Autodesk Fusion 360 part; units mm, degrees
(part 12 of 12)
  arc A2532 (-131.6306, -63.5725) -> (-131.9356, -63.5725) centre (-131.7831, -63.5725) ccw
  arc A2533 (-131.9356, -63.5725) -> (-131.6306, -63.5725) centre (-131.7831, -63.5725) ccw
  arc A2534 (-71.9356, -63.5296) -> (-71.6306, -63.5296) centre (-71.7831, -63.5296) ccw
  arc A2535 (-71.6306, -63.5296) -> (-71.9356, -63.5296) centre (-71.7831, -63.5296) ccw
  arc A2536 (1.2955, -62.3231) -> (0.9905, -62.3231) centre (1.143, -62.3231) ccw
  arc A2537 (0.9905, -62.3231) -> (1.2955, -62.3231) centre (1.143, -62.3231) ccw
  arc A2538 (40.3074, -119.5512) -> (40.0024, -119.5512) centre (40.1549, -119.5512) ccw
  arc A2539 (40.0024, -119.5512) -> (40.3074, -119.5512) centre (40.1549, -119.5512) ccw
  arc A2540 (1.4833, -125.0963) -> (1.7883, -125.0963) centre (1.6358, -125.0963) ccw
  arc A2541 (1.7883, -125.0963) -> (1.4833, -125.0963) centre (1.6358, -125.0963) ccw
  arc A2542 (81.1583, -116.9472) -> (80.8533, -116.9472) centre (81.0058, -116.9472) ccw
  arc A2543 (80.8533, -116.9472) -> (81.1583, -116.9472) centre (81.0058, -116.9472) ccw
  arc A2544 (81.5772, 15.3665) -> (81.8822, 15.3665) centre (81.7297, 15.3665) ccw
  arc A2545 (81.8822, 15.3665) -> (81.5772, 15.3665) centre (81.7297, 15.3665) ccw
  arc A2546 (78.2397, -115.5227) -> (78.5447, -115.5227) centre (78.3922, -115.5227) ccw
  arc A2547 (78.5447, -115.5227) -> (78.2397, -115.5227) centre (78.3922, -115.5227) ccw
  arc A2548 (77.7039, -117.8524) -> (77.3989, -117.8524) centre (77.5514, -117.8524) ccw
  arc A2549 (77.3989, -117.8524) -> (77.7039, -117.8524) centre (77.5514, -117.8524) ccw
  arc A2550 (76.3501, -85.9792) -> (76.0451, -85.9792) centre (76.1976, -85.9792) ccw
  arc A2551 (76.0451, -85.9792) -> (76.3501, -85.9792) centre (76.1976, -85.9792) ccw
  arc A2552 (79.0501, -85.9792) -> (78.7451, -85.9792) centre (78.8976, -85.9792) ccw
  arc A2553 (78.7451, -85.9792) -> (79.0501, -85.9792) centre (78.8976, -85.9792) ccw
  arc A2554 (77.6836, -112.2817) -> (77.3786, -112.2817) centre (77.5311, -112.2817) ccw
  arc A2555 (77.3786, -112.2817) -> (77.6836, -112.2817) centre (77.5311, -112.2817) ccw
  arc A2556 (73.7743, -112.2817) -> (74.0793, -112.2817) centre (73.9268, -112.2817) ccw
  arc A2557 (74.0793, -112.2817) -> (73.7743, -112.2817) centre (73.9268, -112.2817) ccw
  arc A2558 (73.7743, -116.9995) -> (74.0793, -116.9995) centre (73.9268, -116.9995) ccw
  arc A2559 (74.0793, -116.9995) -> (73.7743, -116.9995) centre (73.9268, -116.9995) ccw
  arc A2560 (44.737, -78.1687) -> (45.042, -78.1687) centre (44.8895, -78.1687) ccw
  arc A2561 (45.042, -78.1687) -> (44.737, -78.1687) centre (44.8895, -78.1687) ccw
  arc A2562 (62.8957, -60.3089) -> (62.5907, -60.3089) centre (62.7432, -60.3089) ccw
  arc A2563 (62.5907, -60.3089) -> (62.8957, -60.3089) centre (62.7432, -60.3089) ccw
  arc A2564 (58.0289, -64.1397) -> (58.3339, -64.1397) centre (58.1814, -64.1397) ccw
  arc A2565 (58.3339, -64.1397) -> (58.0289, -64.1397) centre (58.1814, -64.1397) ccw
  arc A2566 (25.4347, -33.4412) -> (25.7398, -33.4412) centre (25.5872, -33.4412) ccw
  arc A2567 (25.7398, -33.4412) -> (25.4347, -33.4412) centre (25.5872, -33.4412) ccw
  arc A2568 (54.4271, -5.5405) -> (54.7321, -5.5405) centre (54.5796, -5.5405) ccw
  arc A2569 (54.7321, -5.5405) -> (54.4271, -5.5405) centre (54.5796, -5.5405) ccw
  arc A2570 (43.932, 19.9916) -> (43.627, 19.9916) centre (43.7795, 19.9916) ccw
  arc A2571 (43.627, 19.9916) -> (43.932, 19.9916) centre (43.7795, 19.9916) ccw
  arc A2572 (30.1477, 19.9916) -> (29.8427, 19.9916) centre (29.9952, 19.9916) ccw
  arc A2573 (29.8427, 19.9916) -> (30.1477, 19.9916) centre (29.9952, 19.9916) ccw
  arc A2574 (54.9582, -6.8923) -> (54.6532, -6.8923) centre (54.8057, -6.8923) ccw
  arc A2575 (54.6532, -6.8923) -> (54.9582, -6.8923) centre (54.8057, -6.8923) ccw
  arc A2576 (19.2295, -34.9096) -> (18.9245, -34.9096) centre (19.077, -34.9096) ccw
  arc A2577 (18.9245, -34.9096) -> (19.2295, -34.9096) centre (19.077, -34.9096) ccw
  arc A2578 (48.9839, -36.415) -> (49.2889, -36.415) centre (49.1364, -36.415) ccw
  arc A2579 (49.2889, -36.415) -> (48.9839, -36.415) centre (49.1364, -36.415) ccw
  arc A2580 (-161.9915, -49.4031) -> (-161.6865, -49.4031) centre (-161.839, -49.4031) ccw
  arc A2581 (-161.6865, -49.4031) -> (-161.9915, -49.4031) centre (-161.839, -49.4031) ccw
  arc A2582 (-178.5523, -46.4056) -> (-178.2473, -46.4056) centre (-178.3998, -46.4056) ccw
  arc A2583 (-178.2473, -46.4056) -> (-178.5523, -46.4056) centre (-178.3998, -46.4056) ccw
  arc A2584 (80.1576, -110.2962) -> (79.8526, -110.2962) centre (80.0051, -110.2962) ccw
  arc A2585 (79.8526, -110.2962) -> (80.1576, -110.2962) centre (80.0051, -110.2962) ccw
  arc A2586 (51.8899, -115.889) -> (51.5849, -115.889) centre (51.7374, -115.889) ccw
  arc A2587 (51.5849, -115.889) -> (51.8899, -115.889) centre (51.7374, -115.889) ccw
  arc A2588 (80.9549, -115.2316) -> (81.2599, -115.2316) centre (81.1074, -115.2316) ccw
  arc A2589 (81.2599, -115.2316) -> (80.9549, -115.2316) centre (81.1074, -115.2316) ccw
  arc A2590 (-184.9643, 17.1631) -> (-185.2693, 17.1631) centre (-185.1168, 17.1631) ccw
  arc A2591 (-185.2693, 17.1631) -> (-184.9643, 17.1631) centre (-185.1168, 17.1631) ccw
  arc A2592 (-169.0275, 17.1631) -> (-168.7225, 17.1631) centre (-168.875, 17.1631) ccw
  arc A2593 (-168.7225, 17.1631) -> (-169.0275, 17.1631) centre (-168.875, 17.1631) ccw
  arc A2594 (45.3849, 16.3147) -> (45.0799, 16.3147) centre (45.2324, 16.3147) ccw
  arc A2595 (45.0799, 16.3147) -> (45.3849, 16.3147) centre (45.2324, 16.3147) ccw
  arc A2596 (68.1408, -38.6081) -> (67.8358, -38.6081) centre (67.9883, -38.6081) ccw
  arc A2597 (67.8358, -38.6081) -> (68.1408, -38.6081) centre (67.9883, -38.6081) ccw
  arc A2598 (-155.29, 20.8895) -> (-155.595, 20.8895) centre (-155.4425, 20.8895) ccw
  arc A2599 (-155.595, 20.8895) -> (-155.29, 20.8895) centre (-155.4425, 20.8895) ccw
  arc A2600 (-124.4523, 23.0592) -> (-124.7573, 23.0592) centre (-124.6048, 23.0592) ccw
  arc A2601 (-124.7573, 23.0592) -> (-124.4523, 23.0592) centre (-124.6048, 23.0592) ccw
  arc A2602 (-121.9328, -27.0211) -> (-122.2378, -27.0211) centre (-122.0853, -27.0211) ccw
  arc A2603 (-122.2378, -27.0211) -> (-121.9328, -27.0211) centre (-122.0853, -27.0211) ccw
  arc A2604 (72.8017, -37.3381) -> (72.4967, -37.3381) centre (72.6492, -37.3381) ccw
  arc A2605 (72.4967, -37.3381) -> (72.8017, -37.3381) centre (72.6492, -37.3381) ccw
  arc A2606 (-90.8551, -43.2421) -> (-91.1601, -43.2421) centre (-91.0076, -43.2421) ccw
  arc A2607 (-91.1601, -43.2421) -> (-90.8551, -43.2421) centre (-91.0076, -43.2421) ccw
  arc A2608 (-88.1108, -46.4056) -> (-87.8058, -46.4056) centre (-87.9583, -46.4056) ccw
  arc A2609 (-87.8058, -46.4056) -> (-88.1108, -46.4056) centre (-87.9583, -46.4056) ccw
  arc A2610 (-67.864, 28.6035) -> (-67.559, 28.6035) centre (-67.7115, 28.6035) ccw
  arc A2611 (-67.559, 28.6035) -> (-67.864, 28.6035) centre (-67.7115, 28.6035) ccw
  arc A2612 (-38.6382, 27.985) -> (-38.9432, 27.985) centre (-38.7907, 27.985) ccw
  arc A2613 (-38.9432, 27.985) -> (-38.6382, 27.985) centre (-38.7907, 27.985) ccw
  arc A2614 (36.2051, -47.3741) -> (35.9001, -47.3741) centre (36.0526, -47.3741) ccw
  arc A2615 (35.9001, -47.3741) -> (36.2051, -47.3741) centre (36.0526, -47.3741) ccw
  arc A2616 (-37.7898, 28.636) -> (-37.4848, 28.636) centre (-37.6373, 28.636) ccw
  arc A2617 (-37.4848, 28.636) -> (-37.7898, 28.636) centre (-37.6373, 28.636) ccw
  arc A2618 (-17.3712, 28.0457) -> (-17.0662, 28.0457) centre (-17.2187, 28.0457) ccw
  arc A2619 (-17.0662, 28.0457) -> (-17.3712, 28.0457) centre (-17.2187, 28.0457) ccw
  arc A2620 (42.4739, -51.3081) -> (42.7789, -51.3081) centre (42.6264, -51.3081) ccw
  arc A2621 (42.7789, -51.3081) -> (42.4739, -51.3081) centre (42.6264, -51.3081) ccw
  arc A2622 (49.9036, -50.0381) -> (49.5986, -50.0381) centre (49.7511, -50.0381) ccw
  arc A2623 (49.5986, -50.0381) -> (49.9036, -50.0381) centre (49.7511, -50.0381) ccw
  arc A2624 (21.1086, 22.5339) -> (20.8036, 22.5339) centre (20.9561, 22.5339) ccw
  arc A2625 (20.8036, 22.5339) -> (21.1086, 22.5339) centre (20.9561, 22.5339) ccw
  arc A2626 (-115.7443, 22.5339) -> (-115.4393, 22.5339) centre (-115.5918, 22.5339) ccw
  arc A2627 (-115.4393, 22.5339) -> (-115.7443, 22.5339) centre (-115.5918, 22.5339) ccw
  arc A2628 (-117.869, 5.461) -> (-117.564, 5.461) centre (-117.7165, 5.461) ccw
  arc A2629 (-117.564, 5.461) -> (-117.869, 5.461) centre (-117.7165, 5.461) ccw
  arc A2630 (-178.0136, 5.461) -> (-177.7086, 5.461) centre (-177.8611, 5.461) ccw
  arc A2631 (-177.7086, 5.461) -> (-178.0136, 5.461) centre (-177.8611, 5.461) ccw
  arc A2632 (68.1307, -73.8407) -> (67.8257, -73.8407) centre (67.9782, -73.8407) ccw
  arc A2633 (67.8257, -73.8407) -> (68.1307, -73.8407) centre (67.9782, -73.8407) ccw
  arc A2634 (76.4972, -73.8407) -> (76.8022, -73.8407) centre (76.6497, -73.8407) ccw
  arc A2635 (76.8022, -73.8407) -> (76.4972, -73.8407) centre (76.6497, -73.8407) ccw
  arc A2636 (77.8462, -114.937) -> (77.5412, -114.937) centre (77.6937, -114.937) ccw
  arc A2637 (77.5412, -114.937) -> (77.8462, -114.937) centre (77.6937, -114.937) ccw
  arc A2638 (-116.4804, -5.8308) -> (-116.1754, -5.8308) centre (-116.3279, -5.8308) ccw
  arc A2639 (-116.1754, -5.8308) -> (-116.4804, -5.8308) centre (-116.3279, -5.8308) ccw
  arc A2640 (-90.2442, -94.2073) -> (-89.9392, -94.2073) centre (-90.0917, -94.2073) ccw
  arc A2641 (-89.9392, -94.2073) -> (-90.2442, -94.2073) centre (-90.0917, -94.2073) ccw
  arc A2642 (-155.29, -9.1105) -> (-155.595, -9.1105) centre (-155.4425, -9.1105) ccw
  arc A2643 (-155.595, -9.1105) -> (-155.29, -9.1105) centre (-155.4425, -9.1105) ccw
  arc A2644 (-124.5213, -6.8494) -> (-124.2163, -6.8494) centre (-124.3688, -6.8494) ccw
  arc A2645 (-124.2163, -6.8494) -> (-124.5213, -6.8494) centre (-124.3688, -6.8494) ccw
  arc A2646 (-148.7294, -6.4173) -> (-149.0344, -6.4173) centre (-148.8819, -6.4173) ccw
  arc A2647 (-149.0344, -6.4173) -> (-148.7294, -6.4173) centre (-148.8819, -6.4173) ccw
  arc A2648 (52.3113, -22.0432) -> (52.6163, -22.0432) centre (52.4638, -22.0432) ccw
  arc A2649 (52.6163, -22.0432) -> (52.3113, -22.0432) centre (52.4638, -22.0432) ccw
  arc A2650 (68.3591, -95.077) -> (68.6641, -95.077) centre (68.5116, -95.077) ccw
  arc A2651 (68.6641, -95.077) -> (68.3591, -95.077) centre (68.5116, -95.077) ccw
  arc A2652 (-126.5478, 2.5314) -> (-126.8528, 2.5314) centre (-126.7003, 2.5314) ccw
  arc A2653 (-126.8528, 2.5314) -> (-126.5478, 2.5314) centre (-126.7003, 2.5314) ccw
  arc A2654 (-95.8876, 2.5314) -> (-95.5826, 2.5314) centre (-95.7351, 2.5314) ccw
  arc A2655 (-95.5826, 2.5314) -> (-95.8876, 2.5314) centre (-95.7351, 2.5314) ccw
  arc A2656 (72.4233, -32.4915) -> (72.1183, -32.4915) centre (72.2708, -32.4915) ccw
  arc A2657 (72.1183, -32.4915) -> (72.4233, -32.4915) centre (72.2708, -32.4915) ccw
  arc A2658 (-64.483, -13.1039) -> (-64.788, -13.1039) centre (-64.6355, -13.1039) ccw
  arc A2659 (-64.788, -13.1039) -> (-64.483, -13.1039) centre (-64.6355, -13.1039) ccw
  arc A2660 (-30.2044, -7.1473) -> (-30.5094, -7.1473) centre (-30.3569, -7.1473) ccw
  arc A2661 (-30.5094, -7.1473) -> (-30.2044, -7.1473) centre (-30.3569, -7.1473) ccw
  arc A2662 (-51.1939, -97.062) -> (-50.8889, -97.062) centre (-51.0414, -97.062) ccw
  arc A2663 (-50.8889, -97.062) -> (-51.1939, -97.062) centre (-51.0414, -97.062) ccw
  arc A2664 (-28.5148, -17.8428) -> (-28.8198, -17.8428) centre (-28.6673, -17.8428) ccw
  arc A2665 (-28.8198, -17.8428) -> (-28.5148, -17.8428) centre (-28.6673, -17.8428) ccw
  arc A2666 (14.0519, -17.8428) -> (13.7469, -17.8428) centre (13.8994, -17.8428) ccw
  arc A2667 (13.7469, -17.8428) -> (14.0519, -17.8428) centre (13.8994, -17.8428) ccw
  arc A2668 (10.6204, -13.8291) -> (10.9254, -13.8291) centre (10.7729, -13.8291) ccw
  arc A2669 (10.9254, -13.8291) -> (10.6204, -13.8291) centre (10.7729, -13.8291) ccw
  arc A2670 (53.6729, -13.8291) -> (53.3679, -13.8291) centre (53.5204, -13.8291) ccw
  arc A2671 (53.3679, -13.8291) -> (53.6729, -13.8291) centre (53.5204, -13.8291) ccw
  arc A2672 (43.4594, -47.7371) -> (43.7644, -47.7371) centre (43.6119, -47.7371) ccw
  arc A2673 (43.7644, -47.7371) -> (43.4594, -47.7371) centre (43.6119, -47.7371) ccw
  arc A2674 (47.3354, -24.9017) -> (47.6404, -24.9017) centre (47.4879, -24.9017) ccw
  arc A2675 (47.6404, -24.9017) -> (47.3354, -24.9017) centre (47.4879, -24.9017) ccw
  arc A2676 (-185.2674, -24.9017) -> (-185.5724, -24.9017) centre (-185.4199, -24.9017) ccw
  arc A2677 (-185.5724, -24.9017) -> (-185.2674, -24.9017) centre (-185.4199, -24.9017) ccw
  arc A2678 (73.6219, -3.683) -> (73.9269, -3.683) centre (73.7744, -3.683) ccw
  arc A2679 (73.9269, -3.683) -> (73.6219, -3.683) centre (73.7744, -3.683) ccw
  arc A2680 (-197.5294, -41.0805) -> (-197.2244, -41.0805) centre (-197.3769, -41.0805) ccw
  arc A2681 (-197.2244, -41.0805) -> (-197.5294, -41.0805) centre (-197.3769, -41.0805) ccw
  arc A2682 (-186.5086, -41.0805) -> (-186.2036, -41.0805) centre (-186.3561, -41.0805) ccw
  arc A2683 (-186.2036, -41.0805) -> (-186.5086, -41.0805) centre (-186.3561, -41.0805) ccw
  arc A2684 (-167.5294, -41.0805) -> (-167.2244, -41.0805) centre (-167.3769, -41.0805) ccw
  arc A2685 (-167.2244, -41.0805) -> (-167.5294, -41.0805) centre (-167.3769, -41.0805) ccw
  arc A2686 (-155.7108, -41.0805) -> (-156.0158, -41.0805) centre (-155.8633, -41.0805) ccw
  arc A2687 (-156.0158, -41.0805) -> (-155.7108, -41.0805) centre (-155.8633, -41.0805) ccw
  arc A2688 (-136.1553, -42.1496) -> (-136.4604, -42.1496) centre (-136.3078, -42.1496) ccw
  arc A2689 (-136.4604, -42.1496) -> (-136.1553, -42.1496) centre (-136.3078, -42.1496) ccw
  arc A2690 (-100.0029, -42.1496) -> (-100.308, -42.1496) centre (-100.1554, -42.1496) ccw
  arc A2691 (-100.308, -42.1496) -> (-100.0029, -42.1496) centre (-100.1554, -42.1496) ccw
  arc A2692 (-107.197, -40.8397) -> (-106.8919, -40.8397) centre (-107.0445, -40.8397) ccw
  arc A2693 (-106.8919, -40.8397) -> (-107.197, -40.8397) centre (-107.0445, -40.8397) ccw
  arc A2694 (-70.069, -40.4031) -> (-70.374, -40.4031) centre (-70.2215, -40.4031) ccw
  arc A2695 (-70.374, -40.4031) -> (-70.069, -40.4031) centre (-70.2215, -40.4031) ccw
  arc A2696 (-78.963, -40.9294) -> (-78.658, -40.9294) centre (-78.8105, -40.9294) ccw
  arc A2697 (-78.658, -40.9294) -> (-78.963, -40.9294) centre (-78.8105, -40.9294) ccw
  arc A2698 (-41.8688, -38.5108) -> (-41.5638, -38.5108) centre (-41.7163, -38.5108) ccw
  arc A2699 (-41.5638, -38.5108) -> (-41.8688, -38.5108) centre (-41.7163, -38.5108) ccw
  arc A2700 (-21.2719, -30.2896) -> (-20.9669, -30.2896) centre (-21.1194, -30.2896) ccw
  arc A2701 (-20.9669, -30.2896) -> (-21.2719, -30.2896) centre (-21.1194, -30.2896) ccw
  arc A2702 (-18.8965, -94.8771) -> (-18.5915, -94.8771) centre (-18.744, -94.8771) ccw
  arc A2703 (-18.5915, -94.8771) -> (-18.8965, -94.8771) centre (-18.744, -94.8771) ccw
  arc A2704 (-42.0182, -40.8832) -> (-42.3232, -40.8832) centre (-42.1707, -40.8832) ccw
  arc A2705 (-42.3232, -40.8832) -> (-42.0182, -40.8832) centre (-42.1707, -40.8832) ccw
  arc A2706 (-12.0804, -38.3053) -> (-11.7754, -38.3053) centre (-11.9279, -38.3053) ccw
  arc A2707 (-11.7754, -38.3053) -> (-12.0804, -38.3053) centre (-11.9279, -38.3053) ccw
  arc A2708 (-49.4223, -27.7981) -> (-49.1172, -27.7981) centre (-49.2697, -27.7981) ccw
  arc A2709 (-49.1172, -27.7981) -> (-49.4223, -27.7981) centre (-49.2697, -27.7981) ccw
  arc A2710 (-41.8785, -99.7239) -> (-42.1835, -99.7239) centre (-42.031, -99.7239) ccw
  arc A2711 (-42.1835, -99.7239) -> (-41.8785, -99.7239) centre (-42.031, -99.7239) ccw
  arc A2712 (62.3926, -99.7239) -> (62.6976, -99.7239) centre (62.5451, -99.7239) ccw
  arc A2713 (62.6976, -99.7239) -> (62.3926, -99.7239) centre (62.5451, -99.7239) ccw
  arc A2714 (42.6976, -30.299) -> (42.3926, -30.299) centre (42.5451, -30.299) ccw
  arc A2715 (42.3926, -30.299) -> (42.6976, -30.299) centre (42.5451, -30.299) ccw
  arc A2716 (15.8695, -42.1496) -> (15.5645, -42.1496) centre (15.717, -42.1496) ccw
  arc A2717 (15.5645, -42.1496) -> (15.8695, -42.1496) centre (15.717, -42.1496) ccw
  arc A2718 (54.9074, -42.031) -> (54.6024, -42.031) centre (54.7549, -42.031) ccw
  arc A2719 (54.6024, -42.031) -> (54.9074, -42.031) centre (54.7549, -42.031) ccw
  arc A2720 (48.0543, -45.4206) -> (48.3593, -45.4206) centre (48.2068, -45.4206) ccw
  arc A2721 (48.3593, -45.4206) -> (48.0543, -45.4206) centre (48.2068, -45.4206) ccw
  arc A2722 (-184.6463, -61.9868) -> (-184.9513, -61.9868) centre (-184.7988, -61.9868) ccw
  arc A2723 (-184.9513, -61.9868) -> (-184.6463, -61.9868) centre (-184.7988, -61.9868) ccw
  arc A2724 (67.7164, -60.1981) -> (68.0214, -60.1981) centre (67.8689, -60.1981) ccw
  arc A2725 (68.0214, -60.1981) -> (67.7164, -60.1981) centre (67.8689, -60.1981) ccw
  arc A2726 (73.8226, -61.257) -> (74.1276, -61.257) centre (73.9751, -61.257) ccw
  arc A2727 (74.1276, -61.257) -> (73.8226, -61.257) centre (73.9751, -61.257) ccw
  arc A2728 (-190.2483, -64.7511) -> (-190.5533, -64.7511) centre (-190.4008, -64.7511) ccw
  arc A2729 (-190.5533, -64.7511) -> (-190.2483, -64.7511) centre (-190.4008, -64.7511) ccw
  arc A2730 (-159.6499, -62.8072) -> (-159.9549, -62.8072) centre (-159.8024, -62.8072) ccw
  arc A2731 (-159.9549, -62.8072) -> (-159.6499, -62.8072) centre (-159.8024, -62.8072) ccw
  arc A2732 (-163.4675, -87.6421) -> (-163.1625, -87.6421) centre (-163.315, -87.6421) ccw
  arc A2733 (-163.1625, -87.6421) -> (-163.4675, -87.6421) centre (-163.315, -87.6421) ccw
  arc A2734 (-117.3039, -62.411) -> (-116.9989, -62.411) centre (-117.1514, -62.411) ccw
  arc A2735 (-116.9989, -62.411) -> (-117.3039, -62.411) centre (-117.1514, -62.411) ccw
  arc A2736 (-99.6494, -62.411) -> (-99.9544, -62.411) centre (-99.8019, -62.411) ccw
  arc A2737 (-99.9544, -62.411) -> (-99.6494, -62.411) centre (-99.8019, -62.411) ccw
  arc A2738 (66.9951, -83.8727) -> (67.3001, -83.8727) centre (67.1476, -83.8727) ccw
  arc A2739 (67.3001, -83.8727) -> (66.9951, -83.8727) centre (67.1476, -83.8727) ccw
  arc A2740 (-54.4495, -83.8839) -> (-54.7545, -83.8839) centre (-54.602, -83.8839) ccw
  arc A2741 (-54.7545, -83.8839) -> (-54.4495, -83.8839) centre (-54.602, -83.8839) ccw
  arc A2742 (4.1754, -84.2367) -> (4.4804, -84.2367) centre (4.3279, -84.2367) ccw
  arc A2743 (4.4804, -84.2367) -> (4.1754, -84.2367) centre (4.3279, -84.2367) ccw
  arc A2744 (-60.9252, -48.7531) -> (-60.6202, -48.7531) centre (-60.7727, -48.7531) ccw
  arc A2745 (-60.6202, -48.7531) -> (-60.9252, -48.7531) centre (-60.7727, -48.7531) ccw
  arc A2746 (51.148, -50.7221) -> (51.453, -50.7221) centre (51.3005, -50.7221) ccw
  arc A2747 (51.453, -50.7221) -> (51.148, -50.7221) centre (51.3005, -50.7221) ccw
  arc A2748 (-32.4619, -57.7719) -> (-32.7669, -57.7719) centre (-32.6144, -57.7719) ccw
  arc A2749 (-32.7669, -57.7719) -> (-32.4619, -57.7719) centre (-32.6144, -57.7719) ccw
  arc A2750 (-7.8797, -57.7719) -> (-7.5747, -57.7719) centre (-7.7272, -57.7719) ccw
  arc A2751 (-7.5747, -57.7719) -> (-7.8797, -57.7719) centre (-7.7272, -57.7719) ccw
  arc A2752 (-51.0245, -111.9929) -> (-50.7195, -111.9929) centre (-50.872, -111.9929) ccw
  arc A2753 (-50.7195, -111.9929) -> (-51.0245, -111.9929) centre (-50.872, -111.9929) ccw
  arc A2754 (-144.1436, -111.9929) -> (-143.8386, -111.9929) centre (-143.9911, -111.9929) ccw
  arc A2755 (-143.8386, -111.9929) -> (-144.1436, -111.9929) centre (-143.9911, -111.9929) ccw
  arc A2756 (3.6204, -52.237) -> (3.3154, -52.237) centre (3.4679, -52.237) ccw
  arc A2757 (3.3154, -52.237) -> (3.6204, -52.237) centre (3.4679, -52.237) ccw
  arc A2758 (-144.6872, -63.5883) -> (-144.9922, -63.5883) centre (-144.8397, -63.5883) ccw
  arc A2759 (-144.9922, -63.5883) -> (-144.6872, -63.5883) centre (-144.8397, -63.5883) ccw
  arc A2760 (55.2605, -86.2377) -> (54.9554, -86.2377) centre (55.108, -86.2377) ccw
  arc A2761 (54.9554, -86.2377) -> (55.2605, -86.2377) centre (55.108, -86.2377) ccw
  arc A2762 (-174.1335, -89.0734) -> (-174.4385, -89.0734) centre (-174.286, -89.0734) ccw
  arc A2763 (-174.4385, -89.0734) -> (-174.1335, -89.0734) centre (-174.286, -89.0734) ccw
  arc A2764 (-147.9285, -84.5438) -> (-148.2335, -84.5438) centre (-148.081, -84.5438) ccw
  arc A2765 (-148.2335, -84.5438) -> (-147.9285, -84.5438) centre (-148.081, -84.5438) ccw
  arc A2766 (53.7796, -85.6949) -> (53.4746, -85.6949) centre (53.6271, -85.6949) ccw
  arc A2767 (53.4746, -85.6949) -> (53.7796, -85.6949) centre (53.6271, -85.6949) ccw
  arc A2768 (-116.3814, -53.2304) -> (-116.6864, -53.2304) centre (-116.5339, -53.2304) ccw
  arc A2769 (-116.6864, -53.2304) -> (-116.3814, -53.2304) centre (-116.5339, -53.2304) ccw
  arc A2770 (-54.9534, -86.4102) -> (-54.6484, -86.4102) centre (-54.8009, -86.4102) ccw
  arc A2771 (-54.6484, -86.4102) -> (-54.9534, -86.4102) centre (-54.8009, -86.4102) ccw
  arc A2772 (-53.9041, -52.8227) -> (-53.5991, -52.8227) centre (-53.7516, -52.8227) ccw
  arc A2773 (-53.5991, -52.8227) -> (-53.9041, -52.8227) centre (-53.7516, -52.8227) ccw
  arc A2774 (23.8465, -52.8227) -> (24.1515, -52.8227) centre (23.999, -52.8227) ccw
  arc A2775 (24.1515, -52.8227) -> (23.8465, -52.8227) centre (23.999, -52.8227) ccw
  arc A2776 (-52.2706, -95.9764) -> (-51.9656, -95.9764) centre (-52.1181, -95.9764) ccw
  arc A2777 (-51.9656, -95.9764) -> (-52.2706, -95.9764) centre (-52.1181, -95.9764) ccw
  arc A2778 (-39.8991, -95.9764) -> (-40.2041, -95.9764) centre (-40.0516, -95.9764) ccw
  arc A2779 (-40.2041, -95.9764) -> (-39.8991, -95.9764) centre (-40.0516, -95.9764) ccw
  arc A2780 (-53.2886, -51.2215) -> (-52.9836, -51.2215) centre (-53.1361, -51.2215) ccw
  arc A2781 (-52.9836, -51.2215) -> (-53.2886, -51.2215) centre (-53.1361, -51.2215) ccw
  arc A2782 (-20.136, -93.1356) -> (-19.831, -93.1356) centre (-19.9835, -93.1356) ccw
  arc A2783 (-19.831, -93.1356) -> (-20.136, -93.1356) centre (-19.9835, -93.1356) ccw
  arc A2784 (1.5701, -93.1356) -> (1.2651, -93.1356) centre (1.4176, -93.1356) ccw
  arc A2785 (1.2651, -93.1356) -> (1.5701, -93.1356) centre (1.4176, -93.1356) ccw
  arc A2786 (-19.9133, -116.5857) -> (-20.2183, -116.5857) centre (-20.0658, -116.5857) ccw
  arc A2787 (-20.2183, -116.5857) -> (-19.9133, -116.5857) centre (-20.0658, -116.5857) ccw
  arc A2788 (-22.9471, -114.5009) -> (-23.2521, -114.5009) centre (-23.0996, -114.5009) ccw
  arc A2789 (-23.2521, -114.5009) -> (-22.9471, -114.5009) centre (-23.0996, -114.5009) ccw
  arc A2790 (-81.7055, -114.5009) -> (-82.0105, -114.5009) centre (-81.858, -114.5009) ccw
  arc A2791 (-82.0105, -114.5009) -> (-81.7055, -114.5009) centre (-81.858, -114.5009) ccw
  arc A2792 (-12.7113, -115.6266) -> (-12.4063, -115.6266) centre (-12.5588, -115.6266) ccw
  arc A2793 (-12.4063, -115.6266) -> (-12.7113, -115.6266) centre (-12.5588, -115.6266) ccw
  arc A2794 (-23.1622, -105.8847) -> (-22.8572, -105.8847) centre (-23.0097, -105.8847) ccw
  arc A2795 (-22.8572, -105.8847) -> (-23.1622, -105.8847) centre (-23.0097, -105.8847) ccw
  arc A2796 (75.8064, -9.034) -> (76.1114, -9.034) centre (75.9589, -9.034) ccw
  arc A2797 (76.1114, -9.034) -> (75.8064, -9.034) centre (75.9589, -9.034) ccw
  arc A2798 (7.0029, -83.224) -> (6.6979, -83.224) centre (6.8504, -83.224) ccw
  arc A2799 (6.6979, -83.224) -> (7.0029, -83.224) centre (6.8504, -83.224) ccw
  arc A2800 (-131.8249, -64.4897) -> (-132.1299, -64.4897) centre (-131.9774, -64.4897) ccw
  arc A2801 (-132.1299, -64.4897) -> (-131.8249, -64.4897) centre (-131.9774, -64.4897) ccw
  arc A2802 (72.5964, 8.4836) -> (72.4765, 8.4836) centre (72.5364, 8.4836) ccw
  arc A2803 (72.4765, 8.4836) -> (72.5964, 8.4836) centre (72.5364, 8.4836) ccw
  arc A2804 (72.506, 4.2926) -> (72.3861, 4.2926) centre (72.446, 4.2926) ccw
  arc A2805 (72.3861, 4.2926) -> (72.506, 4.2926) centre (72.446, 4.2926) ccw
  arc A2806 (-171.4059, 22.7963) -> (-171.286, 22.7963) centre (-171.3459, 22.7963) ccw
  arc A2807 (-171.286, 22.7963) -> (-171.4059, 22.7963) centre (-171.3459, 22.7963) ccw
  arc A2808 (72.4765, 8.4836) -> (72.5964, 8.4836) centre (72.5364, 8.4836) ccw
  arc A2809 (72.5964, 8.4836) -> (72.4765, 8.4836) centre (72.5364, 8.4836) ccw
  arc A2810 (72.3861, 4.2926) -> (72.506, 4.2926) centre (72.446, 4.2926) ccw
  arc A2811 (72.506, 4.2926) -> (72.3861, 4.2926) centre (72.446, 4.2926) ccw
  arc A2812 (-171.4059, 22.7963) -> (-171.286, 22.7963) centre (-171.3459, 22.7963) ccw
  arc A2813 (-171.286, 22.7963) -> (-171.4059, 22.7963) centre (-171.3459, 22.7963) ccw
  arc A2814 (-168.8289, 33.9116) -> (-167.5287, 33.9116) centre (-168.1788, 33.9116) ccw
  arc A2815 (-167.5287, 33.9116) -> (-168.8289, 33.9116) centre (-168.1788, 33.9116) ccw
  arc A2816 (-167.4677, 26.8936) -> (-168.768, 26.8936) centre (-168.1179, 26.8936) ccw
  arc A2817 (-168.768, 26.8936) -> (-167.4677, 26.8936) centre (-168.1179, 26.8936) ccw
  line L1292 (72.9864, 10.0585) -> (72.9864, 8.4835)
  line L1293 (72.5363, 8.4835) -> (72.5363, 10.0585)
  line L1294 (72.5363, 10.0585) -> (72.9864, 10.0585)
  line L1295 (72.9864, 8.4835) -> (72.5363, 8.4835)
  line L1296 (75.1864, 10.0585) -> (75.1864, 8.4835)
  line L1297 (75.6364, 8.4835) -> (75.6364, 10.0585)
  line L1298 (75.6364, 10.0585) -> (75.1864, 10.0585)
  line L1299 (75.1864, 8.4835) -> (75.6364, 8.4835)
  line L1300 (72.4459, 5.8675) -> (72.8959, 5.8675)
  line L1301 (72.4459, 4.2925) -> (72.4459, 5.8675)
  line L1302 (72.8959, 4.2925) -> (72.4459, 4.2925)
  line L1303 (72.8959, 5.8675) -> (72.8959, 4.2925)
  line L1304 (75.5459, 5.8675) -> (75.0959, 5.8675)
  line L1305 (75.0959, 5.8675) -> (75.0959, 4.2925)
  line L1306 (75.0959, 4.2925) -> (75.5459, 4.2925)
  line L1307 (75.5459, 4.2925) -> (75.5459, 5.8675)
  line L1308 (-165.6293, 25.4961) -> (-165.6293, 24.5961)
  line L1309 (-166.3494, 25.4961) -> (-165.6293, 25.4961)
  line L1310 (-165.6293, 24.5961) -> (-166.3494, 24.5961)
  line L1311 (-166.3494, 24.5961) -> (-166.3494, 25.4961)
  line L1312 (-170.7588, 24.4963) -> (-170.0388, 24.4963)
  line L1313 (-170.7588, 23.5961) -> (-170.7588, 24.4963)
  line L1314 (-170.0388, 24.4963) -> (-170.0388, 23.5961)
  line L1315 (-170.0388, 23.5961) -> (-170.7588, 23.5961)
  line L1316 (-166.3494, 28.5961) -> (-166.3494, 29.4961)
  line L1317 (-166.3494, 29.4961) -> (-165.6293, 29.4961)
  line L1318 (-165.6293, 28.5961) -> (-166.3494, 28.5961)
  line L1319 (-165.6293, 29.4961) -> (-165.6293, 28.5961)
  line L1320 (-166.3494, 32.8352) -> (-165.6293, 32.8352)
  line L1321 (-165.6293, 31.935) -> (-166.3494, 31.935)
  line L1322 (-166.3494, 31.935) -> (-166.3494, 32.8352)
  line L1323 (-165.6293, 32.8352) -> (-165.6293, 31.935)
  line L1324 (72.5363, 10.0585) -> (72.9864, 10.0585)
  line L1325 (72.5363, 8.4835) -> (72.5363, 10.0585)
  line L1326 (72.9864, 8.4835) -> (72.5363, 8.4835)
  line L1327 (72.9864, 10.0585) -> (72.9864, 8.4835)
  line L1328 (75.1864, 10.0585) -> (75.1864, 8.4835)
  line L1329 (75.1864, 8.4835) -> (75.6364, 8.4835)
  line L1330 (75.6364, 10.0585) -> (75.1864, 10.0585)
  line L1331 (75.6364, 8.4835) -> (75.6364, 10.0585)
  line L1332 (72.8959, 5.8675) -> (72.8959, 4.2925)
  line L1333 (72.4459, 4.2925) -> (72.4459, 5.8675)
  line L1334 (72.4459, 5.8675) -> (72.8959, 5.8675)
  line L1335 (72.8959, 4.2925) -> (72.4459, 4.2925)
  line L1336 (75.5459, 5.8675) -> (75.0959, 5.8675)
  line L1337 (75.0959, 4.2925) -> (75.5459, 4.2925)
  line L1338 (75.0959, 5.8675) -> (75.0959, 4.2925)
  line L1339 (75.5459, 4.2925) -> (75.5459, 5.8675)
  arc A2818 (-167.5287, 33.9116) -> (-168.8289, 33.9116) centre (-168.1788, 33.9116) ccw
  arc A2819 (-168.8289, 33.9116) -> (-167.5287, 33.9116) centre (-168.1788, 33.9116) ccw
  arc A2820 (-168.768, 26.8936) -> (-167.4677, 26.8936) centre (-168.1179, 26.8936) ccw
  arc A2821 (-167.4677, 26.8936) -> (-168.768, 26.8936) centre (-168.1179, 26.8936) ccw
  line L1340 (-166.3494, 25.4961) -> (-165.6293, 25.4961)
  line L1341 (-165.6293, 24.5961) -> (-166.3494, 24.5961)
  line L1342 (-166.3494, 24.5961) -> (-166.3494, 25.4961)
  line L1343 (-165.6293, 25.4961) -> (-165.6293, 24.5961)
  line L1344 (-170.0388, 24.4963) -> (-170.0388, 23.5961)
  line L1345 (-170.7588, 24.4963) -> (-170.0388, 24.4963)
  line L1346 (-170.0388, 23.5961) -> (-170.7588, 23.5961)
  line L1347 (-170.7588, 23.5961) -> (-170.7588, 24.4963)
  line L1348 (-165.6293, 28.5961) -> (-166.3494, 28.5961)
  line L1349 (-166.3494, 28.5961) -> (-166.3494, 29.4961)
  line L1350 (-165.6293, 29.4961) -> (-165.6293, 28.5961)
  line L1351 (-166.3494, 29.4961) -> (-165.6293, 29.4961)
  line L1352 (-165.6293, 32.8352) -> (-165.6293, 31.935)
  line L1353 (-166.3494, 31.935) -> (-166.3494, 32.8352)
  line L1354 (-165.6293, 31.935) -> (-166.3494, 31.935)
  line L1355 (-166.3494, 32.8352) -> (-165.6293, 32.8352)
  line L1356 (75.6364, 10.0585) -> (75.6364, 8.4835)
  line L1357 (72.5363, 8.4835) -> (72.5363, 10.0585)
  line L1358 (72.5363, 10.0585) -> (75.6364, 10.0585)
  line L1359 (75.6364, 8.4835) -> (72.5363, 8.4835)
  line L1360 (72.4459, 4.2925) -> (72.4459, 5.8675)
  line L1361 (75.5459, 4.2925) -> (72.4459, 4.2925)
  line L1362 (75.5459, 5.8675) -> (75.5459, 4.2925)
  line L1363 (72.4459, 5.8675) -> (75.5459, 5.8675)
  line L1364 (-171.3459, 22.7963) -> (-171.3459, 37.6731)
  line L1365 (-164.9919, 22.7963) -> (-171.3459, 22.7963)
  line L1366 (-164.9919, 37.6731) -> (-164.9919, 22.7963)
  line L1367 (-171.3459, 37.6731) -> (-164.9919, 37.6731)
  line L1368 (72.5363, 8.4835) -> (72.5363, 10.0585)
  line L1369 (75.6364, 8.4835) -> (72.5363, 8.4835)
  line L1370 (75.6364, 10.0585) -> (75.6364, 8.4835)
  line L1371 (72.5363, 10.0585) -> (75.6364, 10.0585)
  line L1372 (72.4459, 4.2925) -> (72.4459, 5.8675)
  line L1373 (75.5459, 5.8675) -> (75.5459, 4.2925)
  line L1374 (72.4459, 5.8675) -> (75.5459, 5.8675)
  line L1375 (75.5459, 4.2925) -> (72.4459, 4.2925)
  line L1376 (-171.3459, 22.7963) -> (-171.3459, 37.6731)
  line L1377 (-171.3459, 37.6731) -> (-164.9919, 37.6731)
  line L1378 (-164.9919, 22.7963) -> (-171.3459, 22.7963)
  line L1379 (-164.9919, 37.6731) -> (-164.9919, 22.7963)
move_body "Move1" bodies 1 to x (1, 0, 0) y (0, 1, 0) z (0, 0, 1) at (-530, -50, 0)
extrude "Extrude2" add sketch "PCB_RIGHT_MAIN" along normal blind 1.5 separate body contours L0 L1 L2 L3 L4 L5 L6 L7 L8 L9 L10 L11 L12 L280 L284 L291 A2806 A2807 A2812 A2813 L1364 L1365 L1366 L1376 L1378 L1379 makes body 2
move_body "Move2" bodies 1 to x (1, 0, 0) y (0, 1, 0) z (0, 0, 1) at (0, 30, 0)
move_body "Move3" bodies 2 to x (1, 0, 0) y (0, 1, 0) z (0, 0, 1) at (0, 30, 0)
move_body "Move4" bodies 2 to x (1, 0, 0) y (0, 1, 0) z (0, 0, 1) at (0, 6, 0)
sketch "Chassis_R" plane through (0, 0, 0) normal (0, 0, 1) x (1, 0, 0)
  line L0 (-198.5014, -46.9312) -> (-198.5014, -71.9502)
  line L1 (-199.5174, -46.9312) -> (-198.5014, -46.9312)
  line L2 (-208.6614, -37.7871) -> (-199.5174, -46.9312)
  line L3 (-198.5014, -71.9502) -> (-214.2494, -87.6982)
  line L4 (-214.2494, -87.6982) -> (-214.2494, -100.0173)
  line L5 (-214.2494, -100.0173) -> (90.1702, -100.0173)
  line L6 (90.1702, -100.0173) -> (90.1702, 73.2111)
  line L7 (90.1702, 73.2111) -> (-164.9919, 73.2111)
  line L8 (-164.9919, 73.2111) -> (-164.9919, 58.7963)
  line L9 (-164.9919, 58.7963) -> (-169.6488, 58.7963)
  line L10 (-171.3459, 58.8563) -> (-171.3459, 73.2111)
  line L11 (-171.3459, 73.2111) -> (-197.4854, 73.2111)
  line L12 (-197.4854, 73.2111) -> (-197.4854, 25.205)
  line L13 (-197.4854, 25.205) -> (-204.5974, 18.093)
  line L14 (-204.5974, 18.093) -> (-208.6614, 18.093)
  line L15 (-208.6614, 18.093) -> (-208.6614, -37.7871)
  line L16 (-171.1488, 63.7963) -> (-171.286, 63.7963)
  line L17 (-166.3459, 78.2111) -> (-169.9919, 78.2111)
  line L18 (-169.9919, 78.2111) -> (-202.4854, 78.2111)
  line L19 (-202.4854, 78.2111) -> (-202.4854, 27.276)
  line L20 (-202.4854, 27.276) -> (-206.6685, 23.093)
  line L21 (-206.6685, 23.093) -> (-213.6614, 23.093)
  line L22 (-213.6614, 23.093) -> (-213.6614, -39.8582)
  line L23 (-213.6614, -39.8582) -> (-203.5014, -50.0182)
  line L24 (-203.5014, -50.0182) -> (-203.5014, -69.8791)
  line L25 (-203.5014, -69.8791) -> (-219.2494, -85.6272)
  line L26 (-219.2494, -85.6272) -> (-219.2494, -105.0173)
  line L27 (-219.2494, -105.0173) -> (95.1702, -105.0173)
  line L28 (95.1702, -105.0173) -> (95.1702, 78.2111)
  line L29 (95.1702, 78.2111) -> (-166.3459, 78.2111)
  line L30 (-171.3459, 58.8563) -> (-171.3459, 58.7964)
  line L31 (-169.6488, 58.7963) -> (-171.3459, 58.7964)
  dimension "d5" = 5
  constraint coincident L10.start L30.start
  constraint coincident L9.end L31.start
sketch "Chassis_L" plane through (0, 0, 0) normal (0, 0, 1) x (1, 0, 0)
  line L0 (-313.3376, -100.6847) -> (-313.3376, -85.9527)
  line L1 (-313.3376, -85.9527) -> (-297.5895, -70.2046)
  line L2 (-297.5895, -70.2046) -> (-297.5895, -45.1856)
  line L3 (-297.5895, -45.1856) -> (-298.6055, -45.1856)
  line L4 (-298.6055, -45.1856) -> (-307.7496, -36.0416)
  line L5 (-307.7496, -36.0416) -> (-307.7496, 19.8386)
  line L6 (-307.7496, 19.8386) -> (-303.6855, 19.8386)
  line L7 (-303.6855, 19.8386) -> (-296.5735, 26.9506)
  line L8 (-296.5735, 26.9506) -> (-296.5735, 72.0357)
  line L9 (-296.5735, 72.0357) -> (-530, 72.0357)
  line L10 (-530, 72.0357) -> (-530, -21.9445)
  line L11 (-530, -21.9445) -> (-529.873, -27.2798)
  line L12 (-529.873, -27.2798) -> (-530, -52.8931)
  line L13 (-530, -52.8931) -> (-530, -101.0262)
  line L14 (-530, -101.0262) -> (-499.7739, -100.6847)
  line L15 (-499.7739, -100.6847) -> (-313.3376, -100.6847)
  line L16 (-302.7496, 14.8386) -> (-301.6145, 14.8386)
  line L17 (-301.6145, 14.8386) -> (-291.5735, 24.8795)
  line L18 (-291.5735, 24.8795) -> (-291.5735, 77.0357)
  line L19 (-291.5735, 77.0357) -> (-535, 77.0357)
  line L20 (-535, 77.0357) -> (-535, -22.004)
  line L21 (-535, -22.004) -> (-534.8733, -27.3269)
  line L22 (-534.8733, -27.3269) -> (-535, -52.8807)
  line L23 (-535, -52.8807) -> (-535, -106.083)
  line L24 (-535, -106.083) -> (-499.7457, -105.6847)
  line L25 (-499.7457, -105.6847) -> (-308.3376, -105.6847)
  line L26 (-308.3376, -105.6847) -> (-308.3376, -88.0237)
  line L27 (-308.3376, -88.0237) -> (-292.5895, -72.2757)
  line L28 (-292.5895, -72.2757) -> (-292.5895, -40.1856)
  line L29 (-292.5895, -40.1856) -> (-296.5345, -40.1856)
  line L30 (-296.5345, -40.1856) -> (-302.7496, -33.9705)
  line L31 (-302.7496, -33.9705) -> (-302.7496, 14.8386)
  dimension "d6" = 5
move_body "Move5" bodies 1 to x (1, 0, 0) y (0, 1, 0) z (0, 0, 1) at (0, 225, 0)
move_body "Move6" bodies 2 to x (1, 0, 0) y (0, 1, 0) z (0, 0, 1) at (0, 225, 0)
extrude "Extrude4" add sketch "Chassis_R" along normal blind 3 separate body contours L0 L1 L2 L3 L4 L5 L6 L7 L8 L9 L10 L11 L12 L13 L14 L15 L30 L31 makes body 3
extrude "Extrude5" add sketch "Chassis_L" along normal blind 3 separate body contours L0 L1 L2 L3 L4 L5 L6 L7 L8 L9 L10 L11 L12 L13 L14 L15 makes body 4
extrude "Extrude6" add sketch "Chassis_R" along normal blind 15 bodies 3
extrude "Extrude7" add sketch "Chassis_L" along normal blind 15 bodies 4
named bodies: "Buildplate_L", "Buildplate_R"
